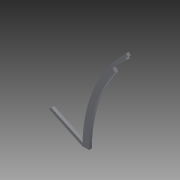
# Autodesk Inventor part: Outer Rail
Saved by Autodesk Inventor 2013 (Build 170138000, 138)
## iProperties
Created: 2013-01-27
Part Number: Outer Rail
Material: Generic
Document SubType Name: Modeling
Designer: Andrew Toennies
Density: 1 g/cm^3
Mass: 13.174 g
Surface Area: 83.7806 cm^2
Volume: 13.174 cm^3
Author: Andrew Toennies
Autodesk Inventor part; units mm, degrees
ref_plane "YZ Plane" through (0, 0, 0) normal (1, 0, 0) x (0, 1, 0)
ref_plane "XZ Plane" through (0, 0, 0) normal (0, 1, 0) x (-1, 0, 0)
ref_plane "XY Plane" through (0, 0, 0) normal (0, 0, 1) x (1, 0, 0)
sketch "Sketch1" plane through (0, 0, 0) normal (0, 0, 1) x (1, 0, 0)
  arc A0 (-220.0163, 220.0163) -> (-311.0719, 6.97) centre (0, 0) ccw
  line L0 (0, 0) -> (-215.5261, 215.5261)
  line L1 (0, 0) -> (-311.15, 0)
  line L2 (-220.0163, 220.0163) -> (-215.5261, 224.5064)
  line L3 (-215.5261, 224.5064) -> (-211.036, 220.0163)
  line L4 (-211.036, 220.0163) -> (-215.5261, 215.5261)
  line L5 (-311.15, 0) -> (-384.6428, 34.2703)
  line L6 (-311.0719, 6.97) -> (-379.8645, 39.0486)
  line L7 (-384.6428, 34.2703) -> (-379.8645, 39.0486)
  arc A1 (-238.9779, 176.1161) -> (-296.8625, 0) centre (0, 0) ccw
  line L8 (-215.5261, 215.5261) -> (-213.2811, 213.2811)
  line L9 (-213.2811, 213.2811) -> (-244.712, 181.8502)
  line L10 (-244.712, 181.8502) -> (-238.9779, 176.1161)
  point P0 (-304.8, 0)
  point P1 (-209.9135, 209.9135)
  dimension "d10" = 45
  dimension "d11" = 6.35
  dimension "d12" = 6.35
  dimension "d13" = 25
  dimension "d14" = 6.35
  dimension "d15" = 76.2
  dimension "d16" = 593.725
  dimension "d18" = 3.175
  dimension "d19" = 44.45
  constraints: 22 end point, 5 point on circle, 4 parallel, 4 point on line, 2 centre point, 2 coincident, 2 perpendicular, 1 horizontal, 1 tangent
  measures "d10" angle of L1 L0
  measures "d11" distance of L2.start L2.end
  measures "d12" distance of L2.end L3.end
  measures "d13" angle of L5 L1
  measures "d14" distance between parallel lines of L6 L5
  measures "d15" distance from line of L1.end L7
  measures "d16" diameter of A1
  measures "d18" distance of L0.end L8.end
  measures "d19" distance of L8.end L9.end
extrude "Extrusion1" add sketch "Sketch1" along normal blind 6.35 contours L2 L3 L4 L0 L9 L10 A1 L1 L5 L7 L6 A0
sketch "Sketch5" plane through (0, 0, 0) normal (0, 0, -1) x (-1, 0, 0)
  line L0 (204.3008, 222.2613) -> (-65.1069, -47.1463) projected
  arc A0 (311.15, 0) -> (220.0163, 220.0163) centre (0, 0) ccw projected
  line L1 (62.8618, 0) -> (311.15, 0) projected
  line L2 (244.712, 181.8502) -> (62.8618, 0) projected
  line L3 (213.2811, 213.2811) -> (244.712, 181.8502) projected
  line L4 (220.0163, 220.0163) -> (213.2811, 213.2811) projected
  circle A1 centre (289.814, 77.6554) radius 1.5875 projected
  circle A2 centre (245.7763, 172.0944) radius 1.5875 projected
  circle A3 centre (303.6401, 26.5651) radius 1.5875 projected
  circle A4 centre (276.2426, 128.814) radius 1.5875 projected
  circle A5 centre (263.9645, 152.4) radius 1.5875 projected
  circle A6 centre (300.1694, 52.928) radius 1.5875 projected
  circle A7 centre (259.8401, 150.0187) radius 1.5875 projected
  circle A8 centre (295.4793, 52.101) radius 1.5875 projected
  circle A9 centre (281.943, 102.6189) radius 1.5875 projected
  circle A10 centre (219.9695, 210.9892) radius 1.5875 projected
  circle A11 centre (286.4183, 104.2477) radius 1.5875 projected
  circle A12 centre (249.6775, 174.8261) radius 1.5875 projected
  circle A13 centre (294.4142, 78.888) radius 1.5875 projected
  circle A14 centre (304.7338, 6.35) radius 1.5875 projected
  circle A15 centre (271.9263, 126.8013) radius 1.5875 projected
  circle A16 centre (298.8958, 26.15) radius 1.5875 projected
extrude "Extrusion2" cut sketch "Sketch5" against normal blind 25.4 contours A1 | A2 | A3 | A4 | A5 | A6 | A7 | A8 | A9 | A11 | A12 | A13 | A14 | A15 | A16
body "Solid1"
